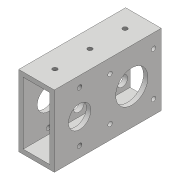
# Autodesk Inventor part: Transmission_Case_ForPrint
Saved by Autodesk Inventor 2018 (Build 220112000, 112)
## iProperties
Created: 2019-08-30
Part Number: Transmission_Case_ForPrint
Material: Generic
Document SubType Name: Modeling
Designer: Clevo
Density: 1 g/cm^3
Appearance: Default
Author: Clevo
Autodesk Inventor part; units mm, degrees
ref_plane "YZ Plane" through (0, 0, 0) normal (1, 0, 0) x (0, 1, 0)
ref_plane "XZ Plane" through (0, 0, 0) normal (0, 1, 0) x (-1, 0, 0)
ref_plane "XY Plane" through (0, 0, 0) normal (0, 0, 1) x (1, 0, 0)
sketch "Sketch1" plane through (0, 0, 0) normal (0, 1, 0) x (-1, 0, 0)
  line L0 (-12.7, 25.4) -> (12.7, 25.4)
  line L1 (12.7, 25.4) -> (12.7, -25.4)
  line L2 (12.7, -25.4) -> (-12.7, -25.4)
  line L3 (-12.7, -25.4) -> (-12.7, 25.4)
  line L4 (-12.7, 25.4) -> (12.7, -25.4) construction
  line L5 (12.7, 25.4) -> (-12.7, -25.4) construction
  point P0 (0, 0)
  dimension "d0" = 50.8
  dimension "d1" = 25.4
  constraints: 12 end point, 2 midpoint, 2 parallel, 1 horizontal, 1 perpendicular
  measures "d0" distance of L0.end L1.end
  measures "d1" distance of L0.start L0.end
extrude "Extrusion1" add sketch "Sketch1" along normal blind 76.2
shell "Shell1" thickness 3.175 removed faces 2 at (-4.2333, 76.2, 8.4667) at (-4.2333, 0, 8.4667)
sketch "Sketch2" plane through (-12.7, 0, -25.4) normal (-1, 0, 0) x (0, 0, 1)
  line L0 (9.9, 39.7) -> (40.9, 39.7)
  line L1 (40.9, 39.7) -> (40.9, 70.7)
  line L2 (40.9, 70.7) -> (9.9, 70.7)
  line L3 (9.9, 70.7) -> (9.9, 39.7)
  line L4 (9.9, 39.7) -> (40.9, 70.7) construction
  line L5 (40.9, 39.7) -> (9.9, 70.7) construction
  line L6 (0, 76.2) -> (50.8, 76.2) projected
  point P0 (25.4, 0)
  point P1 (25.4, 55.2)
  point P2 (25.4, 55.2)
  point P3 (25.4, 76.2)
  dimension "d5" = 31
  dimension "d6" = 31
  dimension "d7" = 21
  constraints: 12 end point, 4 midpoint, 2 parallel, 1 horizontal, 1 perpendicular, 1 vertical alignment
  measures "d5" distance of L1.end L2.end
  measures "d6" distance of L0.end L1.end
  measures "d7" distance from line of L6 point (25.4, 55.2)
hole "Hole1" at (-12.7, 70.7, -15.5) at (-12.7, 70.7, 15.5) at (-12.7, 39.7, 15.5) at (-12.7, 39.7, -15.5) direction (1, 0, 0) diameter 3.2 end through all counterbore diameter 7.5 counterbore depth 5 clearance for "Socket Head Cap Screw" size "M3" standard "Ansi Metric M Profile"
hole "Hole2" at (-12.7, 55.2, 0) direction (1, 0, 0) diameter 10 end through all
sketch "Sketch3" plane through (12.7, 0, 25.4) normal (1, 0, 0) x (0, 0, -1)
  circle A0 centre (25.4, 55.2) radius 5 projected
  circle A1 centre (25.4, 55.2) radius 11.5
  point P0 (25.4, 0)
  dimension "d22" = 23
  constraints: 1 centre point, 1 coincident
  measures "d22" diameter of A1
extrude "Extrusion2" cut sketch "Sketch3" against normal up to surface (22.225 mm away) contours A0 | A1
sketch "Sketch4" plane through (12.7, 0, 25.4) normal (1, 0, 0) x (0, 0, -1)
  circle A0 centre (25.4, 18) radius 8
  line L0 (50.8, 0) -> (0, 0) projected
  point P0 (25.4, 0)
  point P1 (25.4, 0)
  dimension "d25" = 16
  dimension "d26" = 18
  constraints: 1 centre point, 1 midpoint, 1 vertical alignment
  measures "d25" diameter of A0
  measures "d26" distance from line of L0 A0.centre
extrude "Extrusion3" cut sketch "Sketch4" against normal through all
sketch "Sketch6" plane through (12.7, 0, -25.4) normal (0, 0, -1) x (-1, 0, 0)
  line L0 (12.7, 13.1) -> (12.7, 63.1)
  line L1 (25.4, 0) -> (0, 0) projected
  line L2 (0, 76.2) -> (25.4, 76.2) projected
  line L3 (25.4, 0) -> (25.4, 76.2) projected
  point P0 (12.7, 0)
  point P1 (12.7, 38.1)
  point P2 (12.7, 0)
  point P3 (25.4, 38.1)
  dimension "d55" = 50
  constraints: 3 midpoint, 2 end point, 1 horizontal alignment, 1 vertical, 1 vertical alignment
  measures "d55" distance of L0.start L0.end
hole "Hole4" at (0, 38.1, -25.4) at (0, 63.1, -25.4) at (0, 13.1, -25.4) direction (0, 0, 1) diameter 3.242 end through all thread size "M4x0.7" class "6H" standard "ANSI Metric M Profile"
sketch "Sketch7" plane through (12.7, 0, 25.4) normal (1, 0, 0) x (0, 0, -1)
  circle A0 centre (25.4, 18) radius 8 projected
  line L0 (7.4, 18) -> (43.4, 18)
  point P0 (25.4, 0)
  dimension "d47" = 36
  constraints: 2 end point, 1 coincident, 1 horizontal, 1 midpoint
  measures "d47" distance of L0.start L0.end
hole "Hole5" at (12.7, 18, -18) at (12.7, 18, 18) direction (-1, 0, 0) diameter 3.242 end through all thread size "M4x0.7" class "6H" standard "ANSI Metric M Profile"
equation "\"d6\" = d5"
body "Solid1"
